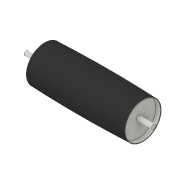
# Autodesk Inventor part: C01
Saved by Autodesk Inventor 2019 (Build 230136000, 136)
## iProperties
Created: 2019-10-31
Part Number: C01
Material: Rubber
Document SubType Name: Modeling
Designer: Carlos Andres garcia velez
Density: 0.93 g/cm^3
Appearance: Rubber - Black
Author: Juan Carlos Botero
Autodesk Inventor part; units mm, degrees
ref_plane "YZ Plane" through (0, 0, 0) normal (1, 0, 0) x (0, 1, 0)
ref_plane "XZ Plane" through (0, 0, 0) normal (0, 1, 0) x (-1, 0, 0)
ref_plane "XY Plane" through (0, 0, 0) normal (0, 0, 1) x (1, 0, 0)
sketch "Sketch1" plane through (0, 0, 0) normal (1, 0, 0) x (0, 1, 0)
  circle A0 centre (0, 0) radius 120
  circle A1 centre (0, 0) radius 117
  dimension "d0" = 240
  dimension "d22" = 3
  constraints: 2 centre point, 2 coincident
  measures "d0" diameter of A0
  measures "d22" radial gap between concentric circles of A1 A0
extrude "Extrusion1" add sketch "Sketch1" along normal mid plane 655
sketch "Sketch2" plane through (0, 0, 0) normal (0, 1, 0) x (-1, 0, 0)
  line L0 (327.5, -120) -> (327.5, 120) projected
  line L1 (327.5, -120) -> (327.5, -122.5)
  line L2 (327.5, -120) -> (-327.5, -120) projected
  line L3 (0, -120) -> (0, -129)
  line L4 (-327.5, -120) -> (-327.5, -122.5)
  arc A0 (-327.5, -122.5) -> (327.5, -122.5) centre (0, 8124.7308) ccw
  line L5 (-327.5, 120) -> (-327.5, -120) projected
  line L6 (327.5, -120) -> (-327.5, -120)
  line L7 (487, 0) -> (-600, 0)
  line L8 (-327.5, -117) -> (327.5, -117) projected
  line L9 (327.5, -117) -> (327.5, -120) projected
  line L10 (-327.5, -120) -> (-327.5, -117) projected
  line L11 (327.5, 117) -> (-327.5, 117) projected
  line L12 (-327.5, 117) -> (-327.5, 120) projected
  line L13 (327.5, 120) -> (327.5, 117) projected
  line L14 (327.5, -120) -> (327.5, 120) projected
  line L15 (-327.5, 120) -> (-327.5, -120) projected
  line L16 (327.5, -120) -> (-327.5, -120) projected
  line L17 (-327.5, 120) -> (327.5, 120) projected
  line L18 (0, -129) -> (-327.5, -129) construction
  line L19 (-327.5, -129) -> (-327.5, -122.5) construction
  point P0 (0, 0)
  dimension "d6" = 2.5
  dimension "d7" = 9
  dimension "d8" = 2.5
  dimension "d10" = 8253.7308
  dimension "d25" = 6.5
  dimension "d27" = 327.5
  constraints: 14 end point, 3 point on circle, 2 horizontal, 2 vertical, 1 centre point, 1 collinear, 1 midpoint, 1 perpendicular, 1 tangent
  measures "d6" distance of L0.start L1.end
  measures "d7" distance of L3.start L3.end
  measures "d8" distance of L2.end L4.end
  measures "d10" radius of A0
  measures "d25" distance of L18.end L4.end
  measures "d27" distance between parallel lines of L4 L3
revolve "Revolution1" add sketch "Sketch2" angle 360 about axis through (-487, 0, 0) along (1, 0, 0) separate body contours L1 A0 L3 L2 | L3 A0 L4 L2
ref_plane "Work Plane1" through (297.5, 0, 0) normal (1, 0, 0) x (0, 0, -1)
sketch "Sketch3" plane through (297.5, 0, 0) normal (1, 0, 0) x (0, 0, -1)
  circle A0 centre (0, 0) radius 117 projected
  circle A1 centre (0, 0) radius 14.2875
  dimension "d26" = 28.575
  constraints: 1 centre point, 1 coincident
  measures "d26" diameter of A1
extrude "Extrusion2" add sketch "Sketch3" against normal blind 3 separate body
ref_plane "Work Plane2" through (-297.5, 0, 0) normal (-1, 0, 0) x (0, 0, 1)
sketch "Sketch4" plane through (-297.5, 0, 0) normal (-1, 0, 0) x (0, 0, 1)
  circle A0 centre (0, 0) radius 117 projected
  circle A1 centre (0, 0) radius 14.2875 projected
extrude "Extrusion3" add sketch "Sketch4" against normal blind 3 separate body
sketch "Sketch5" plane through (-297.5, 0, 0) normal (-1, 0, 0) x (0, 0, 1)
  circle A0 centre (0, 0) radius 14.2875
  dimension "d17" = 28.575
  constraints: 1 centre point, 1 coincident
  measures "d17" diameter of A0
extrude "Extrusion4" add sketch "Sketch5" along normal blind 152 separate body
sketch "Sketch6" plane through (297.5, 0, 0) normal (1, 0, 0) x (0, 0, -1)
  circle A0 centre (0, 0) radius 14.2875 projected
extrude "Extrusion5" add sketch "Sketch6" along normal blind 102 bodies 5
sketch "Sketch7" plane through (-297.5, 0, 0) normal (1, 0, 0) x (0, 0, -1)
  circle A0 centre (0, 0) radius 14.2875 projected
extrude "Extrusion6" add sketch "Sketch7" along normal up to surface (595 mm away) bodies 5
equation "\"d6\" = d8"
body "Solid4"
